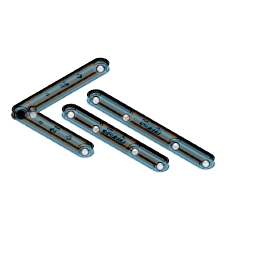
BobsCornerLimitGuidesFUSION (Autodesk Fusion 360 design; units mm, degrees)
Autodesk Fusion 360 part; units mm, degrees
sketch "Sketch1" plane through (0, 0, 0) normal (0, 0, 1) x (1, 0, 0)
  circle A0 centre (0, 0) radius 3.25
  circle A1 centre (128, 0) radius 3.25
  circle A2 centre (0, 159) radius 3.25
  circle A3 centre (0, 159) radius 9
  circle A4 centre (0, 0) radius 9
  circle A5 centre (128, 0) radius 9
  line L0 (-0.0767, -11.9998) -> (128, -12)
  line L1 (-12, 0) -> (-12, 159)
  arc A6 (12, 18.1919) -> (18.1919, 12) centre (12.5, 12.5) ccw
  line L2 (12, 159) -> (12, 18.1919)
  line L3 (18.1919, 12) -> (128, 12)
  arc A7 (128, -12) -> (128, 12) centre (128, 0) ccw
  arc A8 (12, 159) -> (-12, 159) centre (0, 159) ccw
  arc A9 (8.851, 8.1031) -> (8.1031, 8.851) centre (0, 0) ccw
  arc A10 (-12, 0) -> (0.0767, -11.9998) centre (0, 0) ccw
  line L4 (-0.0701, -9.9998) -> (128, -10)
  arc A11 (128, -10) -> (128, 10) centre (128, 0) ccw
  line L5 (19.7975, 10) -> (128, 10)
  arc A12 (10, 19.7975) -> (19.7975, 10) centre (12.5, 12.5) ccw
  line L6 (10, 159) -> (10, 19.7975)
  arc A13 (10, 159) -> (-10, 159) centre (0, 159) ccw
  line L7 (-10, 0) -> (-10, 159)
  arc A14 (-10, 0) -> (-0.0701, -9.9998) centre (0, 0) ccw
  dimension "d1" = 6.5
  dimension "d2" = 159
  dimension "d3" = 128
  dimension "d4" = 6.5
  dimension "d5" = 6.5
  dimension "d6" = 18
  dimension "d7" = 18
  dimension "d8" = 18
  dimension "d9" = 24
  dimension "d10" = 24
  dimension "d11" = 24
  dimension "d18" = 2
  constraint coincident A0.centre A4.centre
  constraint concentric A2 A3
  constraint concentric A1 A7
  constraint concentric A4 A9
  constraint concentric A3 A8
  constraint coincident L0.start A9
  constraint tangent L0 A7
  constraint tangent L2 A9
  constraint coincident L1.start A9
  constraint tangent L1 A8
  constraint vertical L1
  constraint tangent L3 A7
  constraint perpendicular L2 L3
  constraint coincident L0 A10.end
  constraint coincident A6 A9.start
  constraint coincident A6 A9.end
  constraint concentric A9 A10
  measures "d1" diameter of A0
  measures "d2" distance of A0.centre A2.centre
  measures "d3" distance of A0.centre A1.centre
  measures "d4" diameter of A1
  measures "d5" diameter of A2
  measures "d6" diameter of A3
  measures "d7" diameter of A4
  measures "d8" diameter of A5
  measures "d9" diameter of A7
  measures "d10" diameter of A9
  measures "d11" diameter of A8
extrude "Extrude3" add sketch "Sketch1" along normal blind 10 contours L0 L1 A6 L2 L3 A7 A8 A10 makes body 1
extrude "Extrude4" add sketch "Sketch1" along normal blind 8 contours L4 A11 L5 A12 L6 A13 L7 A14 bodies 1
extrude "Extrude5" add sketch "Sketch1" along normal blind 3.2 contours A3 | A4 | A5 bodies 1
sketch "Sketch4" plane through (0, 0, 8) normal (0, 0, 1) x (-1, 0, 0)
  circle A0 centre (-128, 0) radius 9
  circle A1 centre (0, 0) radius 9
  circle A2 centre (0, -159) radius 9
  arc A3 (-10, -159) -> (10, -159) centre (0, -159) ccw
  line L0 (10, -159) -> (10, 0)
  arc A4 (10, 0) -> (0.0701, 9.9998) centre (0, 0) ccw
  line L1 (0.0701, 9.9998) -> (-128, 10)
  arc A5 (-128, 10) -> (-128, -10) centre (-128, 0) ccw
  line L2 (-128, -10) -> (-19.7975, -10)
  arc A6 (-10, -19.7975) -> (-19.7975, -10) centre (-12.5, -12.5) ccw
  line L3 (-10, -19.7975) -> (-10, -159)
  line L4 (10, -19.7975) -> (-10, -19.7975) construction
  line L5 (-10, -19.7975) -> (-10, -150) construction
  line L6 (-10, -150) -> (10, -150) construction
  line L7 (10, -150) -> (10, -19.7975) construction
  line L8 (-19.9362, 9.9998) -> (-120.0403, 9.9998) construction
  line L9 (-120.0403, 9.9998) -> (-120.0403, -10) construction
  line L10 (-120.0403, -10) -> (-19.9362, -10) construction
  line L11 (-19.9362, -10) -> (-19.9362, 9.9998) construction
  dimension "d25" = 10
  dimension "d26" = 10
  text T0 "+\n\nY\n\n-" font "Arial" height 10 bold align centre middle in box 20 x 130.2025 at (10, -19.7975) x (-1, 0) y (0, -1) spacing 1 kerned
  text T1 "-     X     +" font "Arial" height 10 bold align centre middle in box 100.1041 x 19.9998 at (-19.9362, 9.9998) x (-1, 0) y (0, -1) spacing 1 kerned
  constraint coincident A6.start
  constraint coincident L0
  constraint coincident L1
  constraint coincident L2
sketch "Sketch9" plane through (0, 0, 0) normal (0, 0, 1) x (1, 0, 0)
  line L0 (49.9605, 61.9999) -> (228, 62)
  line L1 (228, 38) -> (50, 38)
  line L2 (50.0021, 112) -> (269, 112)
  line L3 (269, 88) -> (50, 88)
  arc A0 (50.0021, 112) -> (50, 88) centre (50, 100) ccw
  arc A1 (110.0018, 112) -> (109.9982, 112) centre (110, 100) ccw
  arc A2 (209.0011, 112) -> (208.9989, 112) centre (209, 100) ccw
  arc A3 (269, 88) -> (269, 112) centre (269, 100) ccw
  arc A4 (228, 38) -> (228, 62) centre (228, 50) ccw
  arc A5 (178.0209, 62) -> (177.9791, 62) centre (178, 50) ccw
  arc A6 (100.0335, 62) -> (99.9665, 62) centre (100, 50) ccw
  arc A7 (50.0395, 61.9999) -> (50, 38) centre (50, 50) ccw
  line L4 (49.951, 53.1746) -> (50.049, 53.1746)
  arc A8 (50.049, 53.1746) -> (49.951, 53.1746) centre (50, 50) ccw
  arc A9 (269, 90) -> (269, 110) centre (269, 100) ccw
  line L5 (50.0011, 110) -> (269, 110)
  arc A10 (50.0011, 110) -> (50, 90) centre (50, 100) ccw
  line L6 (269, 90) -> (50, 90)
  line L7 (49.9639, 59.9999) -> (228, 60)
  arc A11 (228, 40) -> (228, 60) centre (228, 50) ccw
  line L8 (228, 40) -> (50, 40)
  arc A12 (49.9639, 59.9999) -> (50, 40) centre (50, 50) ccw
  circle A13 centre (50, 100) radius 3.25
  circle A14 centre (110, 100) radius 3.25
  line L9 (50, 109) -> (110, 109)
  line L10 (110, 91) -> (50, 91)
  arc A15 (50, 109) -> (50, 91) centre (50, 100) ccw
  arc A16 (110, 91) -> (110, 109) centre (110, 100) ccw
  circle A17 centre (209, 100) radius 3.25
  circle A18 centre (269, 100) radius 3.25
  line L11 (269, 91) -> (209, 91)
  line L12 (209, 109) -> (269, 109)
  arc A19 (209, 109) -> (209, 91) centre (209, 100) ccw
  arc A20 (269, 91) -> (269, 109) centre (269, 100) ccw
  circle A21 centre (50, 50) radius 3.25
  circle A22 centre (100, 50) radius 3.25
  line L13 (100, 59) -> (50, 59)
  line L14 (50, 41) -> (100, 41)
  arc A23 (50, 59) -> (50, 41) centre (50, 50) ccw
  arc A24 (100, 41) -> (100, 59) centre (100, 50) ccw
  circle A25 centre (228, 50) radius 3.25
  circle A26 centre (178, 50) radius 3.25
  line L15 (178, 59) -> (228, 59)
  line L16 (228, 41) -> (178, 41)
  arc A27 (178, 59) -> (178, 41) centre (178, 50) ccw
  arc A28 (228, 41) -> (228, 59) centre (228, 50) ccw
  dimension "d83" = 24
  dimension "d97" = 2
  dimension "d98" = 2
  dimension "d109" = 6.5
  dimension "d110" = 18
  dimension "d111" = 6.5
  dimension "d112" = 18
  dimension "d113" = 6.5
  dimension "d114" = 6.5
  dimension "d115" = 18
  dimension "d116" = 18
  dimension "d117" = 6.5
  dimension "d118" = 6.5
  dimension "d120" = 18
  dimension "d121" = 18
  dimension "d122" = 6.5
  dimension "d123" = 6.5
  dimension "d124" = 18
  dimension "d125" = 18
  constraint coincident L0.start A7
  constraint tangent L0 A4
  constraint tangent L1 A7
  constraint horizontal L1
  constraint tangent L2 A3
  constraint tangent L3 A0
  constraint horizontal L3
  constraint coincident L2 A1.end
  constraint coincident L2 A1.start
  constraint coincident L2 A2.end
  constraint coincident L2 A2.start
  constraint coincident L0 A5.start
  constraint coincident L0 A5.end
  constraint coincident L0 A6.start
  constraint coincident L0 A6.end
  constraint coincident L0 A7.start
  constraint concentric A0 A13
  constraint concentric A13 A15
  constraint concentric A1 A14
  constraint concentric A1 A16
  constraint tangent L9 A16
  constraint tangent L10 A15
  constraint parallel L6 L10
  constraint concentric A3 A18
  constraint concentric A17 A19
  constraint concentric A18 A20
  constraint tangent L11 A19
  constraint parallel L6 L11
  constraint tangent L12 A20
  constraint horizontal L12
  constraint concentric A7 A21
  constraint concentric A6 A24
  constraint concentric A8 A23
  constraint tangent L13 A23
  constraint horizontal L13
  constraint tangent L14 A24
  constraint parallel L8 L14
  constraint concentric A4 A25
  constraint concentric A5 A26
  constraint concentric A26 A27
  constraint concentric A4 A28
  constraint tangent L15 A28
  constraint horizontal L15
  constraint tangent L16 A27
  constraint parallel L8 L16
  measures "d83" diameter of A3
  measures "d109" diameter of A13
  measures "d110" diameter of A15
  measures "d111" diameter of A14
  measures "d112" diameter of A16
  measures "d113" diameter of A17
  measures "d114" diameter of A18
  measures "d115" diameter of A19
  measures "d116" diameter of A20
  measures "d117" diameter of A21
  measures "d118" diameter of A22
  measures "d120" diameter of A24
  measures "d121" diameter of A23
  measures "d122" diameter of A25
  measures "d123" diameter of A26
  measures "d124" diameter of A27
  measures "d125" diameter of A28
extrude "Extrude11" add sketch "Sketch9" along normal blind 10 separate body contours L0 L1 A4 A5 A6 A7 | L2 L3 A0 A1 A2 A3 makes body 2 at (196, 90, 3.3333) makes body 3 at (109.3093, 60, 3.3333)
extrude "Extrude15" add sketch "Sketch9" along normal blind 8 contours A9 L5 A10 L6 | L7 A11 L8 A12 bodies 2 3
extrude "Extrude16" add sketch "Sketch9" along normal blind 3.2 contours L9 L10 A15 A16 | L11 L12 A19 A20 | L13 L14 A23 A24 | L15 L16 A27 A28 bodies 2 3
sketch "Sketch11" plane through (0, 0, 8) normal (0, 0, 1) x (-1, 0, 0)
  arc A0 (-209, -109) -> (-209, -91) centre (-209, -100) ccw
  line L0 (-209, -109) -> (-269, -109)
  arc A1 (-269, -91) -> (-269, -109) centre (-269, -100) ccw
  line L1 (-269, -91) -> (-209, -91)
  arc A2 (-50, -109) -> (-50, -91) centre (-50, -100) ccw
  line L2 (-50, -109) -> (-110, -109)
  arc A3 (-110, -91) -> (-110, -109) centre (-110, -100) ccw
  line L3 (-110, -91) -> (-50, -91)
  arc A4 (-50.0011, -110) -> (-50, -90) centre (-50, -100) ccw
  line L4 (-50, -90) -> (-269, -90)
  arc A5 (-269, -90) -> (-269, -110) centre (-269, -100) ccw
  line L5 (-269, -110) -> (-50.0011, -110)
  line L6 (-119, -90) -> (-199.9246, -90) construction
  line L7 (-199.9246, -90) -> (-199.9246, -110) construction
  line L8 (-199.9246, -110) -> (-119, -110) construction
  line L9 (-119, -110) -> (-119, -90) construction
  line L10 (-109, -40) -> (-169, -40) construction
  line L11 (-169, -40) -> (-169, -60) construction
  line L12 (-169, -60) -> (-109, -60) construction
  line L13 (-109, -60) -> (-109, -40) construction
  dimension "d130" = 10
  dimension "d131" = 10
  text T0 "Y-axis" font "Arial" height 10 bold align centre middle in box 80.9246 x 20 at (-119, -90) x (-1, 0) y (0, -1) spacing 1 kerned
  text T1 "X-axis" font "Arial" height 10 bold align centre middle in box 60 x 20 at (-109, -40) x (-1, 0) y (0, -1) spacing 1 kerned
  constraint coincident L4
  constraint coincident L5
extrude "Extrude17" add sketch "Sketch11" along normal blind 2 text T1 T0 bodies 2 3
extrude "Extrude18" add sketch "Sketch4" along normal blind 2 text T1 T0 bodies 1
